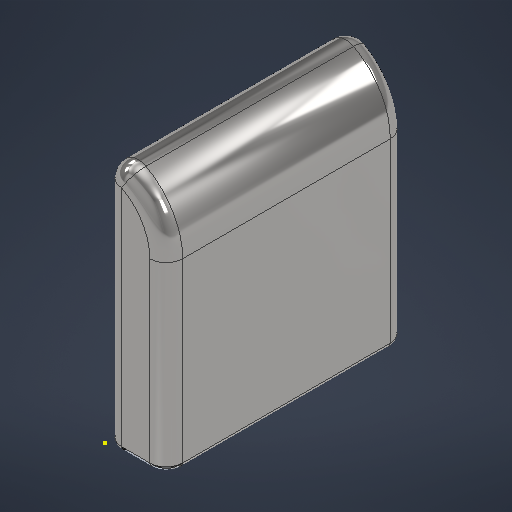
# Autodesk Inventor part: chairbase
Saved by Autodesk Inventor 2027 (Build 310192000, 192)
## iProperties
Created: 2026-04-24
Part Number: chairbase
Material: Sherpa
Document SubType Name: Modeling
Designer: sisis
Density: 0.9 g/cm^3
Appearance: Shepra
Author: sisis
Autodesk Inventor part; units mm, degrees
ref_plane "YZ Plane" through (0, 0, 0) normal (1, 0, 0) x (0, 1, 0)
ref_plane "XZ Plane" through (0, 0, 0) normal (0, 1, 0) x (-1, 0, 0)
ref_plane "XY Plane" through (0, 0, 0) normal (0, 0, 1) x (1, 0, 0)
sketch "Sketch1" plane through (0, 0, 0) normal (0, 1, 0) x (-1, 0, 0)
  point P0 (0, 0)
sketch "Sketch2" plane through (0, 0, 0) normal (1, 0, 0) x (0, 1, 0)
  line L0 (0, 0) -> (13.614, 0)
  line L1 (13.614, 0) -> (13.614, -13.0302)
  line L2 (13.614, -13.0302) -> (0, -13.0302)
  line L3 (0, -13.0302) -> (0, 0)
  dimension "d23" = 13.0302
  constraints: 8 end point, 3 perpendicular, 1 horizontal
  measures "d23" distance of L0.end L1.end
extrude "Extrusion1" add sketch "Sketch2" along normal blind 3.302
fillet "Fillet1" radius 3.81 1 edges at (3.302, 13.614, -6.5151)
sketch "Sketch3" plane through (0, 0, -13.0302) normal (0, -1, 0) x (1, 0, 0)
  circle A0 centre (1.4178, 10.266) radius 0.8102
  circle A1 centre (1.4178, 2.7686) radius 0.8102
  line L0 (0, 13.0302) -> (3.302, 13.0302) projected
  line L1 (0, 0) -> (3.302, 0) projected
  line L2 (0, 13.0302) -> (0, 0) projected
  point P0 (1.651, 13.0302)
  point P1 (1.651, 0)
  dimension "d17" = 1.6204
  dimension "d18" = 2.7642
  dimension "d19" = 2.7686
  dimension "d20" = 1.4178
  dimension "d21" = 1.6204
  dimension "d22" = 1.4178
  constraints: 2 centre point, 2 midpoint
  measures "d17" diameter of A1
  measures "d18" vertical distance of point (1.651, 13.03) A0.centre
  measures "d19" vertical distance of point (1.651, 0) A1.centre
  measures "d20" distance from line of L2 A0.centre
  measures "d21" diameter of A0
  measures "d22" distance from line of A1.centre L2
extrude "Extrusion2" add sketch "Sketch3" along normal blind 0.635
sketch "Sketch4" plane through (0, 0, 0) normal (-1, 0, 0) x (0, 0, 1)
  circle A0 centre (-2.2352, 11.6328) radius 0.7112
  circle A1 centre (-2.2352, 1.9812) radius 0.7112
  circle A2 centre (-10.795, 1.9812) radius 0.7112
  circle A3 centre (-10.795, 11.6328) radius 0.7112
  line L0 (0, 13.614) -> (0, 0) projected
  line L1 (0, 0) -> (-13.0302, 0) projected
  line L2 (-13.0302, 0) -> (-13.0302, 13.614) projected
  line L3 (-13.0302, 13.614) -> (0, 13.614) projected
  dimension "d9" = 1.4224
  dimension "d12" = 1.4224
  dimension "d13" = 1.4224
  dimension "d14" = 1.4224
  dimension "d25" = 1.524
  dimension "d26" = 1.27
  dimension "d27" = 1.27
  dimension "d28" = 1.524
  dimension "d29" = 1.524
  dimension "d30" = 1.524
  dimension "d31" = 1.27
  dimension "d32" = 1.27
  dimension "d33" = 7.1374
  dimension "d34" = 7.1374
  dimension "d35" = 8.2292
  dimension "d36" = 8.2292
  constraints: 4 centre point
  measures "d9" diameter of A0
  measures "d12" diameter of A1
  measures "d13" diameter of A2
  measures "d14" diameter of A3
  measures "d25" distance edge to line of A1 L0
  measures "d26" distance edge to line of A1 L1
  measures "d27" distance edge to line of A2 L1
  measures "d28" distance edge to line of A2 L2
  measures "d29" distance edge to line of A3 L2
  measures "d30" distance edge to line of A0 L0
  measures "d31" distance edge to line of A3 L3
  measures "d32" distance edge to line of A0 L3
extrude "Extrusion3" cut sketch "Sketch4" against normal blind 1.27 contours A0 | A1 | A2 | A3
fillet "Fillet2" radius 0.889 1 edges at (0, 13.614, -6.5151)
fillet "Fillet3" radius 0.889 4 edges at (0, 6.2016, -13.0302) (0.4349, 13.1676, -13.0302) (2.7676, 11.784, -13.0302) (3.302, 4.919, -13.0302)
fillet "Fillet4" radius 0.889 4 edges at (0, 6.2016, 0) (0.4349, 13.1676, 0) (2.7676, 11.784, 0) (3.302, 4.919, 0)
fillet "Fillet5" radius 0.254 8 edges at (3.302, 0, -6.5151) (3.0416, 0, -12.7698) (1.651, 0, -13.0302) (0.2604, 0, -12.7698) (0, 0, -6.5151) (0.2604, 0, -0.2604) (1.651, 0, 0) (3.0416, 0, -0.2604)
body "Solid1"
